Autodesk Fusion 360 part; units mm, degrees
(part 5 of 15)
sketch "Sketch1" plane through (0, 0, 0) normal (0, 0, 1) x (1, 0, 0) in component "Component"
  spline S0 degree 5 poles (15.0052, -0.9615) (15.0053, -0.9615) (15.0055, -0.9615) (15.0058, -0.9615) (15.0063, -0.9616) (15.0071, -0.9616) (15.008, -0.9616) (15.0091, -0.9617) (15.0102, -0.9617) (15.0115, -0.9618) (15.0128, -0.9618) (15.0143, -0.9619) (15.0159, -0.9619) (15.0176, -0.9619) (15.0194, -0.962) (15.0213, -0.962) (15.0234, -0.962) (15.0255, -0.9621) (15.0277, -0.9621) (15.0301, -0.9621) (15.0325, -0.9621) (15.0351, -0.9621) (15.0377, -0.9621) (15.0404, -0.9621) (15.0433, -0.9621) (15.0462, -0.9621) (15.0492, -0.962) (15.0523, -0.962) (15.0555, -0.9619) (15.0588, -0.9619) (15.0622, -0.9618) (15.0657, -0.9617) (15.0693, -0.9616) (15.0729, -0.9615) (15.0767, -0.9614) (15.0805, -0.9612) (15.0844, -0.9611) (15.0884, -0.9609) (15.0925, -0.9607) (15.0967, -0.9606) (15.1009, -0.9603) (15.1053, -0.9601) (15.1097, -0.9599) (15.1142, -0.9596) (15.1187, -0.9594) (15.1234, -0.9591) (15.1281, -0.9588) (15.1329, -0.9585) (15.1378, -0.9581) (15.1427, -0.9578) (15.1477, -0.9574) (15.1528, -0.957) (15.158, -0.9566) (15.1633, -0.9562) (15.1686, -0.9558) (15.174, -0.9553) (15.1794, -0.9548) (15.1849, -0.9543) (15.1905, -0.9538) (15.1962, -0.9533) (15.2019, -0.9527) (15.2077, -0.9521) (15.2136, -0.9515) (15.2196, -0.9509) (15.2256, -0.9503) (15.2316, -0.9496) (15.2378, -0.9489) (15.244, -0.9482) (15.2502, -0.9475) (15.2565, -0.9467) (15.2629, -0.946) (15.2694, -0.9452) (15.2759, -0.9444) (15.2825, -0.9435) (15.2891, -0.9427) (15.2958, -0.9418) (15.3025, -0.9408) (15.3094, -0.9399) (15.3162, -0.9389) (15.3232, -0.938) (15.3301, -0.937) (15.3372, -0.9359) (15.3443, -0.9349) (15.3515, -0.9338) (15.3587, -0.9327) (15.3659, -0.9315) (15.3733, -0.9304) (15.3807, -0.9292) (15.3881, -0.928) (15.3956, -0.9267) (15.4031, -0.9255) (15.4107, -0.9242) (15.4184, -0.9229) (15.4261, -0.9215) (15.4338, -0.9202) (15.4417, -0.9188) (15.4495, -0.9173) (15.4574, -0.9159) (15.4654, -0.9144) (15.4734, -0.9129) (15.4815, -0.9114) (15.4896, -0.9098) (15.4977, -0.9082) (15.5059, -0.9066) (15.5142, -0.905) (15.5225, -0.9033) (15.5309, -0.9016) (15.5393, -0.8999) (15.5477, -0.8981) (15.5562, -0.8963) (15.5648, -0.8945) (15.5733, -0.8927) (15.582, -0.8908) (15.5907, -0.8889) (15.5994, -0.887) (15.6081, -0.885) (15.617, -0.883) (15.6258, -0.881) (15.6347, -0.879) (15.6437, -0.8769) (15.6527, -0.8748) (15.6617, -0.8726) (15.6708, -0.8705) (15.6799, -0.8683) (15.689, -0.866) (15.6982, -0.8638) (15.7075, -0.8615) (15.7168, -0.8592) (15.7261, -0.8568) (15.7354, -0.8544) (15.7448, -0.852) (15.7543, -0.8496) (15.7638, -0.8471) (15.7733, -0.8446) (15.7829, -0.8421) (15.7925, -0.8395) (15.8021, -0.8369) (15.8118, -0.8343) (15.8215, -0.8316) (15.8313, -0.8289) (15.841, -0.8262) (15.8509, -0.8235) (15.8607, -0.8207) (15.8706, -0.8178) (15.8806, -0.815) (15.8906, -0.8121) (15.9006, -0.8092) (15.9106, -0.8063) (15.9207, -0.8033) (15.9308, -0.8003) (15.941, -0.7972) (15.9512, -0.7941) (15.9614, -0.791) (15.9716, -0.7879) (15.9819, -0.7847) (15.9923, -0.7815) (16.0026, -0.7783) (16.013, -0.775) (16.0234, -0.7717) (16.0339, -0.7683) (16.0444, -0.765) (16.0549, -0.7616) (16.0655, -0.7581) (16.0761, -0.7547) (16.0867, -0.7512) (16.0973, -0.7476) (16.108, -0.744) (16.1187, -0.7404) (16.1295, -0.7368) (16.1402, -0.7331) (16.151, -0.7294) (16.1619, -0.7257) (16.1727, -0.7219) (16.1836, -0.7181) (16.1946, -0.7143) (16.2055, -0.7104) (16.2165, -0.7065) (16.2275, -0.7025) (16.2385, -0.6986) (16.2496, -0.6946) (16.2607, -0.6905) (16.2718, -0.6864) (16.283, -0.6823) (16.2942, -0.6782) (16.3054, -0.674) (16.3166, -0.6698) (16.3279, -0.6655) (16.3391, -0.6612) (16.3505, -0.6569) (16.3618, -0.6526) (16.3732, -0.6482) (16.3846, -0.6438) (16.396, -0.6393) (16.4074, -0.6348) (16.4189, -0.6303) (16.4304, -0.6257) (16.4419, -0.6211) (16.4535, -0.6165) (16.465, -0.6118) (16.4766, -0.6071) (16.4882, -0.6024) (16.4999, -0.5976) (16.5116, -0.5928) (16.5233, -0.588) (16.535, -0.5831) (16.5467, -0.5782) (16.5585, -0.5732) (16.5703, -0.5683) (16.5821, -0.5632) (16.5939, -0.5582) (16.6057, -0.5531) (16.6176, -0.548) (16.6295, -0.5428) (16.6414, -0.5376) (16.6534, -0.5324) (16.6653, -0.5271) (16.6773, -0.5218) (16.6893, -0.5165) (16.7014, -0.5111) (16.7134, -0.5057) (16.7255, -0.5003) (16.7376, -0.4948) (16.7497, -0.4893) (16.7618, -0.4837) (16.774, -0.4782) (16.7861, -0.4725) (16.7983, -0.4669) (16.8105, -0.4612) (16.8228, -0.4555) (16.835, -0.4497) (16.8473, -0.4439) (16.8596, -0.4381) (16.8719, -0.4322) (16.8842, -0.4263) (16.8965, -0.4203) (16.9089, -0.4144) (16.9213, -0.4084) (16.9337, -0.4023) (16.9461, -0.3962) (16.9585, -0.3901) (16.971, -0.3839) (16.981, -0.379) (16.9884, -0.3753) (16.9934, -0.3728) (16.9959, -0.3715) knots 0 0 0 0 0 0 0.00416667 0.00833333 0.0125 0.01666667 0.02083333 0.025 0.02916667 0.03333333 0.0375 0.04166667 0.04583333 0.05 0.05416667 0.05833333 0.0625 0.06666667 0.07083333 0.075 0.07916667 0.08333333 0.0875 0.09166667 0.09583333 0.1 0.10416667 0.10833333 0.1125 0.11666667 0.12083333 0.125 0.12916667 0.13333333 0.1375 0.14166667 0.14583333 0.15 0.15416667 0.15833333 0.1625 0.16666667 0.17083333 0.175 0.17916667 0.18333333 0.1875 0.19166667 0.19583333 0.2 0.20416667 0.20833333 0.2125 0.21666667 0.22083333 0.225 0.22916667 0.23333333 0.2375 0.24166667 0.24583333 0.25 0.25416667 0.25833333 0.2625 0.26666667 0.27083333 0.275 0.27916667 0.28333333 0.2875 0.29166667 0.29583333 0.3 0.30416667 0.30833333 0.3125 0.31666667 0.32083333 0.325 0.32916667 0.33333333 0.3375 0.34166667 0.34583333 0.35 0.35416667 0.35833333 0.3625 0.36666667 0.37083333 0.375 0.37916667 0.38333333 0.3875 0.39166667 0.39583333 0.4 0.40416667 0.40833333 0.4125 0.41666667 0.42083333 0.425 0.42916667 0.43333333 0.4375 0.44166667 0.44583333 0.45 0.45416667 0.45833333 0.4625 0.46666667 0.47083333 0.475 0.47916667 0.48333333 0.4875 0.49166667 0.49583333 0.5 0.50416667 0.50833333 0.5125 0.51666667 0.52083333 0.525 0.52916667 0.53333333 0.5375 0.54166667 0.54583333 0.55 0.55416667 0.55833333 0.5625 0.56666667 0.57083333 0.575 0.57916667 0.58333333 0.5875 0.59166667 0.59583333 0.6 0.60416667 0.60833333 0.6125 0.61666667 0.62083333 0.625 0.62916667 0.63333333 0.6375 0.64166667 0.64583333 0.65 0.65416667 0.65833333 0.6625 0.66666667 0.67083333 0.675 0.67916667 0.68333333 0.6875 0.69166667 0.69583333 0.7 0.70416667 0.70833333 0.7125 0.71666667 0.72083333 0.725 0.72916667 0.73333333 0.7375 0.74166667 0.74583333 0.75 0.75416667 0.75833333 0.7625 0.76666667 0.77083333 0.775 0.77916667 0.78333333 0.7875 0.79166667 0.79583333 0.8 0.80416667 0.80833333 0.8125 0.81666667 0.82083333 0.825 0.82916667 0.83333333 0.8375 0.84166667 0.84583333 0.85 0.85416667 0.85833333 0.8625 0.86666667 0.87083333 0.875 0.87916667 0.88333333 0.8875 0.89166667 0.89583333 0.9 0.90416667 0.90833333 0.9125 0.91666667 0.92083333 0.925 0.92916667 0.93333333 0.9375 0.94166667 0.94583333 0.95 0.95416667 0.95833333 0.9625 0.96666667 0.97083333 0.975 0.97916667 0.98333333 0.9875 0.99166667 0.99583333 1 1 1 1 1 1
  spline S1 degree 5 poles (15.0052, 0.9615) (15.0053, 0.9615) (15.0055, 0.9615) (15.0058, 0.9615) (15.0063, 0.9616) (15.0071, 0.9616) (15.008, 0.9616) (15.0091, 0.9617) (15.0102, 0.9617) (15.0115, 0.9618) (15.0128, 0.9618) (15.0143, 0.9619) (15.0159, 0.9619) (15.0176, 0.9619) (15.0194, 0.962) (15.0213, 0.962) (15.0234, 0.962) (15.0255, 0.9621) (15.0277, 0.9621) (15.0301, 0.9621) (15.0325, 0.9621) (15.0351, 0.9621) (15.0377, 0.9621) (15.0404, 0.9621) (15.0433, 0.9621) (15.0462, 0.9621) (15.0492, 0.962) (15.0523, 0.962) (15.0555, 0.9619) (15.0588, 0.9619) (15.0622, 0.9618) (15.0657, 0.9617) (15.0693, 0.9616) (15.0729, 0.9615) (15.0767, 0.9614) (15.0805, 0.9612) (15.0844, 0.9611) (15.0884, 0.9609) (15.0925, 0.9607) (15.0967, 0.9606) (15.1009, 0.9603) (15.1053, 0.9601) (15.1097, 0.9599) (15.1142, 0.9596) (15.1187, 0.9594) (15.1234, 0.9591) (15.1281, 0.9588) (15.1329, 0.9585) (15.1378, 0.9581) (15.1427, 0.9578) (15.1477, 0.9574) (15.1528, 0.957) (15.158, 0.9566) (15.1633, 0.9562) (15.1686, 0.9558) (15.174, 0.9553) (15.1794, 0.9548) (15.1849, 0.9543) (15.1905, 0.9538) (15.1962, 0.9533) (15.2019, 0.9527) (15.2077, 0.9521) (15.2136, 0.9515) (15.2196, 0.9509) (15.2256, 0.9503) (15.2316, 0.9496) (15.2378, 0.9489) (15.244, 0.9482) (15.2502, 0.9475) (15.2565, 0.9467) (15.2629, 0.946) (15.2694, 0.9452) (15.2759, 0.9444) (15.2825, 0.9435) (15.2891, 0.9427) (15.2958, 0.9418) (15.3025, 0.9408) (15.3094, 0.9399) (15.3162, 0.9389) (15.3232, 0.938) (15.3301, 0.937) (15.3372, 0.9359) (15.3443, 0.9349) (15.3515, 0.9338) (15.3587, 0.9327) (15.3659, 0.9315) (15.3733, 0.9304) (15.3807, 0.9292) (15.3881, 0.928) (15.3956, 0.9267) (15.4031, 0.9255) (15.4107, 0.9242) (15.4184, 0.9229) (15.4261, 0.9215) (15.4338, 0.9202) (15.4417, 0.9188) (15.4495, 0.9173) (15.4574, 0.9159) (15.4654, 0.9144) (15.4734, 0.9129) (15.4815, 0.9114) (15.4896, 0.9098) (15.4977, 0.9082) (15.5059, 0.9066) (15.5142, 0.905) (15.5225, 0.9033) (15.5309, 0.9016) (15.5393, 0.8999) (15.5477, 0.8981) (15.5562, 0.8963) (15.5648, 0.8945) (15.5733, 0.8927) (15.582, 0.8908) (15.5907, 0.8889) (15.5994, 0.887) (15.6081, 0.885) (15.617, 0.883) (15.6258, 0.881) (15.6347, 0.879) (15.6437, 0.8769) (15.6527, 0.8748) (15.6617, 0.8726) (15.6708, 0.8705) (15.6799, 0.8683) (15.689, 0.866) (15.6982, 0.8638) (15.7075, 0.8615) (15.7168, 0.8592) (15.7261, 0.8568) (15.7354, 0.8544) (15.7448, 0.852) (15.7543, 0.8496) (15.7638, 0.8471) (15.7733, 0.8446) (15.7829, 0.8421) (15.7925, 0.8395) (15.8021, 0.8369) (15.8118, 0.8343) (15.8215, 0.8316) (15.8313, 0.8289) (15.841, 0.8262) (15.8509, 0.8235) (15.8607, 0.8207) (15.8706, 0.8178) (15.8806, 0.815) (15.8906, 0.8121) (15.9006, 0.8092) (15.9106, 0.8063) (15.9207, 0.8033) (15.9308, 0.8003) (15.941, 0.7972) (15.9512, 0.7941) (15.9614, 0.791) (15.9716, 0.7879) (15.9819, 0.7847) (15.9923, 0.7815) (16.0026, 0.7783) (16.013, 0.775) (16.0234, 0.7717) (16.0339, 0.7683) (16.0444, 0.765) (16.0549, 0.7616) (16.0655, 0.7581) (16.0761, 0.7547) (16.0867, 0.7512) (16.0973, 0.7476) (16.108, 0.744) (16.1187, 0.7404) (16.1295, 0.7368) (16.1402, 0.7331) (16.151, 0.7294) (16.1619, 0.7257) (16.1727, 0.7219) (16.1836, 0.7181) (16.1946, 0.7143) (16.2055, 0.7104) (16.2165, 0.7065) (16.2275, 0.7025) (16.2385, 0.6986) (16.2496, 0.6946) (16.2607, 0.6905) (16.2718, 0.6864) (16.283, 0.6823) (16.2942, 0.6782) (16.3054, 0.674) (16.3166, 0.6698) (16.3279, 0.6655) (16.3391, 0.6612) (16.3505, 0.6569) (16.3618, 0.6526) (16.3732, 0.6482) (16.3846, 0.6438) (16.396, 0.6393) (16.4074, 0.6348) (16.4189, 0.6303) (16.4304, 0.6257) (16.4419, 0.6211) (16.4535, 0.6165) (16.465, 0.6118) (16.4766, 0.6071) (16.4882, 0.6024) (16.4999, 0.5976) (16.5116, 0.5928) (16.5233, 0.588) (16.535, 0.5831) (16.5467, 0.5782) (16.5585, 0.5732) (16.5703, 0.5683) (16.5821, 0.5632) (16.5939, 0.5582) (16.6057, 0.5531) (16.6176, 0.548) (16.6295, 0.5428) (16.6414, 0.5376) (16.6534, 0.5324) (16.6653, 0.5271) (16.6773, 0.5218) (16.6893, 0.5165) (16.7014, 0.5111) (16.7134, 0.5057) (16.7255, 0.5003) (16.7376, 0.4948) (16.7497, 0.4893) (16.7618, 0.4837) (16.774, 0.4782) (16.7861, 0.4725) (16.7983, 0.4669) (16.8105, 0.4612) (16.8228, 0.4555) (16.835, 0.4497) (16.8473, 0.4439) (16.8596, 0.4381) (16.8719, 0.4322) (16.8842, 0.4263) (16.8965, 0.4203) (16.9089, 0.4144) (16.9213, 0.4084) (16.9337, 0.4023) (16.9461, 0.3962) (16.9585, 0.3901) (16.971, 0.3839) (16.981, 0.379) (16.9884, 0.3753) (16.9934, 0.3728) (16.9959, 0.3715) knots 0 0 0 0 0 0 0.00416667 0.00833333 0.0125 0.01666667 0.02083333 0.025 0.02916667 0.03333333 0.0375 0.04166667 0.04583333 0.05 0.05416667 0.05833333 0.0625 0.06666667 0.07083333 0.075 0.07916667 0.08333333 0.0875 0.09166667 0.09583333 0.1 0.10416667 0.10833333 0.1125 0.11666667 0.12083333 0.125 0.12916667 0.13333333 0.1375 0.14166667 0.14583333 0.15 0.15416667 0.15833333 0.1625 0.16666667 0.17083333 0.175 0.17916667 0.18333333 0.1875 0.19166667 0.19583333 0.2 0.20416667 0.20833333 0.2125 0.21666667 0.22083333 0.225 0.22916667 0.23333333 0.2375 0.24166667 0.24583333 0.25 0.25416667 0.25833333 0.2625 0.26666667 0.27083333 0.275 0.27916667 0.28333333 0.2875 0.29166667 0.29583333 0.3 0.30416667 0.30833333 0.3125 0.31666667 0.32083333 0.325 0.32916667 0.33333333 0.3375 0.34166667 0.34583333 0.35 0.35416667 0.35833333 0.3625 0.36666667 0.37083333 0.375 0.37916667 0.38333333 0.3875 0.39166667 0.39583333 0.4 0.40416667 0.40833333 0.4125 0.41666667 0.42083333 0.425 0.42916667 0.43333333 0.4375 0.44166667 0.44583333 0.45 0.45416667 0.45833333 0.4625 0.46666667 0.47083333 0.475 0.47916667 0.48333333 0.4875 0.49166667 0.49583333 0.5 0.50416667 0.50833333 0.5125 0.51666667 0.52083333 0.525 0.52916667 0.53333333 0.5375 0.54166667 0.54583333 0.55 0.55416667 0.55833333 0.5625 0.56666667 0.57083333 0.575 0.57916667 0.58333333 0.5875 0.59166667 0.59583333 0.6 0.60416667 0.60833333 0.6125 0.61666667 0.62083333 0.625 0.62916667 0.63333333 0.6375 0.64166667 0.64583333 0.65 0.65416667 0.65833333 0.6625 0.66666667 0.67083333 0.675 0.67916667 0.68333333 0.6875 0.69166667 0.69583333 0.7 0.70416667 0.70833333 0.7125 0.71666667 0.72083333 0.725 0.72916667 0.73333333 0.7375 0.74166667 0.74583333 0.75 0.75416667 0.75833333 0.7625 0.76666667 0.77083333 0.775 0.77916667 0.78333333 0.7875 0.79166667 0.79583333 0.8 0.80416667 0.80833333 0.8125 0.81666667 0.82083333 0.825 0.82916667 0.83333333 0.8375 0.84166667 0.84583333 0.85 0.85416667 0.85833333 0.8625 0.86666667 0.87083333 0.875 0.87916667 0.88333333 0.8875 0.89166667 0.89583333 0.9 0.90416667 0.90833333 0.9125 0.91666667 0.92083333 0.925 0.92916667 0.93333333 0.9375 0.94166667 0.94583333 0.95 0.95416667 0.95833333 0.9625 0.96666667 0.97083333 0.975 0.97916667 0.98333333 0.9875 0.99166667 0.99583333 1 1 1 1 1 1
  spline S2 degree 5 poles (15.0043, -0.9615) (15.0043, -0.9615) (15.0044, -0.9615) (15.0045, -0.9615) (15.0047, -0.9615) (15.0048, -0.9615) (15.005, -0.9615) (15.0051, -0.9615) (15.0051, -0.9615) (15.0052, -0.9615) knots 0 0 0 0 0 0 0.2 0.4 0.6 0.8 1 1 1 1 1 1
  spline S3 degree 5 poles (15.0043, 0.9615) (15.0043, 0.9615) (15.0044, 0.9615) (15.0045, 0.9615) (15.0047, 0.9615) (15.0048, 0.9615) (15.005, 0.9615) (15.0051, 0.9615) (15.0051, 0.9615) (15.0052, 0.9615) knots 0 0 0 0 0 0 0.2 0.4 0.6 0.8 1 1 1 1 1 1
  line L0 (0, 0) -> (15.0043, -0.9615)
  line L1 (0, 0) -> (15.0043, 0.9615)
  arc A0 (16.9959, -0.3715) -> (16.9959, 0.3715) centre (0, 0) ccw
  point P0 (15.0078, -0.9616)
  point P1 (15.0121, -0.9618)
  point P2 (15.0182, -0.962)
  point P3 (15.0261, -0.9621)
  point P4 (15.0357, -0.9621)
  point P5 (15.047, -0.9621)
  point P6 (15.0601, -0.9618)
  point P7 (15.0749, -0.9614)
  point P8 (15.0915, -0.9608)
  point P9 (15.1097, -0.9599)
  point P10 (15.1298, -0.9587)
  point P11 (15.1515, -0.9571)
  point P12 (15.175, -0.9552)
  point P13 (15.2001, -0.9529)
  point P14 (15.227, -0.9501)
  point P15 (15.2556, -0.9469)
  point P16 (15.2859, -0.9431)
  point P17 (15.3179, -0.9387)
  point P18 (15.3515, -0.9338)
  point P19 (15.3868, -0.9282)
  point P20 (15.4238, -0.9219)
  point P21 (15.4624, -0.915)
  point P22 (15.5026, -0.9073)
  point P23 (15.5445, -0.8988)
  point P24 (15.588, -0.8895)
  point P25 (15.6331, -0.8793)
  point P26 (15.6797, -0.8683)
  point P27 (15.728, -0.8563)
  point P28 (15.7777, -0.8434)
  point P29 (15.8291, -0.8295)
  point P30 (15.8819, -0.8146)
  point P31 (15.9363, -0.7986)
  point P32 (15.9922, -0.7815)
  point P33 (16.0495, -0.7633)
  point P34 (16.1083, -0.7439)
  point P35 (16.1685, -0.7234)
  point P36 (16.2302, -0.7016)
  point P37 (16.2932, -0.6785)
  point P38 (16.3576, -0.6542)
  point P39 (16.4234, -0.6285)
  point P40 (16.4905, -0.6014)
  point P41 (16.559, -0.573)
  point P42 (16.6287, -0.5432)
  point P43 (16.6997, -0.5119)
  point P44 (16.772, -0.4791)
  point P45 (16.8454, -0.4448)
  point P46 (16.9201, -0.4089)
  point P47 (15.0078, 0.9616)
  point P48 (15.0121, 0.9618)
  point P49 (15.0182, 0.962)
  point P50 (15.0261, 0.9621)
  point P51 (15.0357, 0.9621)
  point P52 (15.047, 0.9621)
  point P53 (15.0601, 0.9618)
  point P54 (15.0749, 0.9614)
  point P55 (15.0915, 0.9608)
  point P56 (15.1097, 0.9599)
  point P57 (15.1298, 0.9587)
  point P58 (15.1515, 0.9571)
  point P59 (15.175, 0.9552)
  point P60 (15.2001, 0.9529)
  point P61 (15.227, 0.9501)
  point P62 (15.2556, 0.9469)
  point P63 (15.2859, 0.9431)
  point P64 (15.3179, 0.9387)
  point P65 (15.3515, 0.9338)
  point P66 (15.3868, 0.9282)
  point P67 (15.4238, 0.9219)
  point P68 (15.4624, 0.915)
  point P69 (15.5026, 0.9073)
  point P70 (15.5445, 0.8988)
  point P71 (15.588, 0.8895)
  point P72 (15.6331, 0.8793)
  point P73 (15.6797, 0.8683)
  point P74 (15.728, 0.8563)
  point P75 (15.7777, 0.8434)
  point P76 (15.8291, 0.8295)
  point P77 (15.8819, 0.8146)
  point P78 (15.9363, 0.7986)
  point P79 (15.9922, 0.7815)
  point P80 (16.0495, 0.7633)
  point P81 (16.1083, 0.7439)
  point P82 (16.1685, 0.7234)
  point P83 (16.2302, 0.7016)
  point P84 (16.2932, 0.6785)
  point P85 (16.3576, 0.6542)
  point P86 (16.4234, 0.6285)
  point P87 (16.4905, 0.6014)
  point P88 (16.559, 0.573)
  point P89 (16.6287, 0.5432)
  point P90 (16.6997, 0.5119)
  point P91 (16.772, 0.4791)
  point P92 (16.8454, 0.4448)
  point P93 (16.9201, 0.4089)
sketch "Sketch2" plane through (0, 0, 0) normal (0, 0, 1) x (1, 0, 0) in component "Component"
  circle A0 centre (0, 0) radius 14.75
extrude "Extrude1" add sketch "Sketch2" along normal blind 10 makes body 1 in component "Component"
extrude "Extrude2" add sketch "Sketch1" along normal blind 10 separate body makes body 2 in component "Component"
pattern_circular "C-Pattern1" count 32 over 360 about axis through (0, 0, 1.75) along (0, 0, 1) of "Extrude2" makes body 3 at (4.8431, 1.2901, 3.3333) makes body 4 at (4.7436, 1.618, 3.3333) makes body 5 at (4.3368, 2.5123, 3.3333) makes body 6 at (3.7634, 3.3101, 6.6667) makes body 7 at (3.0453, 3.9807, 3.3333) makes body 8 at (2.2102, 4.4983, 6.6667) makes body 9 at (1.2901, 4.8431, 3.3333) makes body 10 at (0.3205, 5.0017, 3.3333) makes body 11 at (-1.2901, 4.8431, 3.3333) makes body 12 at (-1.618, 4.7436, 6.6667) makes body 13 at (-2.5123, 4.3368, 3.3333) makes body 14 at (-3.3101, 3.7634, 3.3333) makes body 15 at (-3.9807, 3.0453, 3.3333) makes body 16 at (-4.7436, 1.618, 3.3333) makes body 17 at (-4.8431, 1.2901, 3.3333) makes body 18 at (-5.0017, 0.3205, 6.6667) makes body 19 at (-4.9681, -0.6614, 6.6667) makes body 20 at (-4.7436, -1.618, 6.6667) makes body 21 at (-4.3368, -2.5123, 3.3333) makes body 22 at (-3.7634, -3.3101, 3.3333) makes body 23 at (-3.0453, -3.9807, 3.3333) makes body 24 at (-2.2102, -4.4983, 3.3333) makes body 25 at (-1.2901, -4.8431, 3.3333) makes body 26 at (-0.3205, -5.0017, 6.6667) makes body 27 at (0.6614, -4.9681, 6.6667) makes body 28 at (1.618, -4.7436, 6.6667) makes body 29 at (2.5123, -4.3368, 3.3333) makes body 30 at (3.3101, -3.7634, 6.6667) makes body 31 at (4.3368, -2.5123, 3.3333) makes body 32 at (4.7436, -1.618, 6.6667) makes body 33 at (4.8431, -1.2901, 3.3333) in component "Component"
combine "Combine1" operation add target body 1 tool bodies 2 3 4 5 6 7 8 9 10 11 12 13 14 15 16 17 18 19 20 21 22 23 24 25 26 27 28 29 30 31 32 33 in component "Component"
sketch "Sketch3" plane through (0, 0, 0) normal (0, 0, 1) x (1, 0, 0) in component "Component"
  line L0 (0, 0) -> (47.0171, 0) construction
  line L1 (47.0171, 0) -> (47.0171, 3) construction
  line L2 (47.0171, 3) -> (0, 3) construction
  line L3 (0, 3) -> (0, 0) construction
  constraint perpendicular L0 L1
  constraint parallel L0 L2
  constraint parallel L1 L3
sketch "Sketch1 (2)" plane through (0, 0, 10) normal (0, 0, 1) x (-1, 0, 0)
  arc A0 (-14.621, 1.9466) -> (-14.7198, 0.9432) centre (0, 0) ccw
  line L0 (-14.7198, 0.9432) -> (-15.0043, 0.9615)
  line L1 (-15.0043, 0.9615) -> (-15.0052, 0.9615)
  spline S0 degree 5 poles (-15.0052, 0.9615) (-15.0053, 0.9615) (-15.0055, 0.9615) (-15.0058, 0.9615) (-15.0063, 0.9616) (-15.0071, 0.9616) (-15.008, 0.9616) (-15.0091, 0.9617) (-15.0102, 0.9617) (-15.0115, 0.9618) (-15.0128, 0.9618) (-15.0143, 0.9619) (-15.0159, 0.9619) (-15.0176, 0.9619) (-15.0194, 0.962) (-15.0213, 0.962) (-15.0234, 0.962) (-15.0255, 0.9621) (-15.0277, 0.9621) (-15.0301, 0.9621) (-15.0325, 0.9621) (-15.0351, 0.9621) (-15.0377, 0.9621) (-15.0404, 0.9621) (-15.0433, 0.9621) (-15.0462, 0.9621) (-15.0492, 0.962) (-15.0523, 0.962) (-15.0555, 0.9619) (-15.0588, 0.9619) (-15.0622, 0.9618) (-15.0657, 0.9617) (-15.0693, 0.9616) (-15.0729, 0.9615) (-15.0767, 0.9614) (-15.0805, 0.9612) (-15.0844, 0.9611) (-15.0884, 0.9609) (-15.0925, 0.9607) (-15.0967, 0.9606) (-15.1009, 0.9603) (-15.1053, 0.9601) (-15.1097, 0.9599) (-15.1142, 0.9596) (-15.1187, 0.9594) (-15.1234, 0.9591) (-15.1281, 0.9588) (-15.1329, 0.9585) (-15.1378, 0.9581) (-15.1427, 0.9578) (-15.1477, 0.9574) (-15.1528, 0.957) (-15.158, 0.9566) (-15.1633, 0.9562) (-15.1686, 0.9558) (-15.174, 0.9553) (-15.1794, 0.9548) (-15.1849, 0.9543) (-15.1905, 0.9538) (-15.1962, 0.9533) (-15.2019, 0.9527) (-15.2077, 0.9521) (-15.2136, 0.9515) (-15.2196, 0.9509) (-15.2256, 0.9503) (-15.2316, 0.9496) (-15.2378, 0.9489) (-15.244, 0.9482) (-15.2502, 0.9475) (-15.2565, 0.9467) (-15.2629, 0.946) (-15.2694, 0.9452) (-15.2759, 0.9444) (-15.2825, 0.9435) (-15.2891, 0.9427) (-15.2958, 0.9418) (-15.3025, 0.9408) (-15.3094, 0.9399) (-15.3162, 0.9389) (-15.3232, 0.938) (-15.3301, 0.937) (-15.3372, 0.9359) (-15.3443, 0.9349) (-15.3515, 0.9338) (-15.3587, 0.9327) (-15.3659, 0.9315) (-15.3733, 0.9304) (-15.3807, 0.9292) (-15.3881, 0.928) (-15.3956, 0.9267) (-15.4031, 0.9255) (-15.4107, 0.9242) (-15.4184, 0.9229) (-15.4261, 0.9215) (-15.4338, 0.9202) (-15.4417, 0.9188) (-15.4495, 0.9173) (-15.4574, 0.9159) (-15.4654, 0.9144) (-15.4734, 0.9129) (-15.4815, 0.9114) (-15.4896, 0.9098) (-15.4977, 0.9082) (-15.5059, 0.9066) (-15.5142, 0.905) (-15.5225, 0.9033) (-15.5309, 0.9016) (-15.5393, 0.8999) (-15.5477, 0.8981) (-15.5562, 0.8963) (-15.5648, 0.8945) (-15.5733, 0.8927) (-15.582, 0.8908) (-15.5907, 0.8889) (-15.5994, 0.887) (-15.6081, 0.885) (-15.617, 0.883) (-15.6258, 0.881) (-15.6347, 0.879) (-15.6437, 0.8769) (-15.6527, 0.8748) (-15.6617, 0.8726) (-15.6708, 0.8705) (-15.6799, 0.8683) (-15.689, 0.866) (-15.6982, 0.8638) (-15.7075, 0.8615) (-15.7168, 0.8592) (-15.7261, 0.8568) (-15.7354, 0.8544) (-15.7448, 0.852) (-15.7543, 0.8496) (-15.7638, 0.8471) (-15.7733, 0.8446) (-15.7829, 0.8421) (-15.7925, 0.8395) (-15.8021, 0.8369) (-15.8118, 0.8343) (-15.8215, 0.8316) (-15.8313, 0.8289) (-15.841, 0.8262) (-15.8509, 0.8235) (-15.8607, 0.8207) (-15.8706, 0.8178) (-15.8806, 0.815) (-15.8906, 0.8121) (-15.9006, 0.8092) (-15.9106, 0.8063) (-15.9207, 0.8033) (-15.9308, 0.8003) (-15.941, 0.7972) (-15.9512, 0.7941) (-15.9614, 0.791) (-15.9716, 0.7879) (-15.9819, 0.7847) (-15.9923, 0.7815) (-16.0026, 0.7783) (-16.013, 0.775) (-16.0234, 0.7717) (-16.0339, 0.7683) (-16.0444, 0.765) (-16.0549, 0.7616) (-16.0655, 0.7581) (-16.0761, 0.7547) (-16.0867, 0.7512) (-16.0973, 0.7476) (-16.108, 0.744) (-16.1187, 0.7404) (-16.1295, 0.7368) (-16.1402, 0.7331) (-16.151, 0.7294) (-16.1619, 0.7257) (-16.1727, 0.7219) (-16.1836, 0.7181) (-16.1946, 0.7143) (-16.2055, 0.7104) (-16.2165, 0.7065) (-16.2275, 0.7025) (-16.2385, 0.6986) (-16.2496, 0.6946) (-16.2607, 0.6905) (-16.2718, 0.6864) (-16.283, 0.6823) (-16.2942, 0.6782) (-16.3054, 0.674) (-16.3166, 0.6698) (-16.3279, 0.6655) (-16.3391, 0.6612) (-16.3505, 0.6569) (-16.3618, 0.6526) (-16.3732, 0.6482) (-16.3846, 0.6438) (-16.396, 0.6393) (-16.4074, 0.6348) (-16.4189, 0.6303) (-16.4304, 0.6257) (-16.4419, 0.6211) (-16.4535, 0.6165) (-16.465, 0.6118) (-16.4766, 0.6071) (-16.4882, 0.6024) (-16.4999, 0.5976) (-16.5116, 0.5928) (-16.5233, 0.588) (-16.535, 0.5831) (-16.5467, 0.5782) (-16.5585, 0.5732) (-16.5703, 0.5683) (-16.5821, 0.5632) (-16.5939, 0.5582) (-16.6057, 0.5531) (-16.6176, 0.548) (-16.6295, 0.5428) (-16.6414, 0.5376) (-16.6534, 0.5324) (-16.6653, 0.5271) (-16.6773, 0.5218) (-16.6893, 0.5165) (-16.7014, 0.5111) (-16.7134, 0.5057) (-16.7255, 0.5003) (-16.7376, 0.4948) (-16.7497, 0.4893) (-16.7618, 0.4837) (-16.774, 0.4782) (-16.7861, 0.4725) (-16.7983, 0.4669) (-16.8105, 0.4612) (-16.8228, 0.4555) (-16.835, 0.4497) (-16.8473, 0.4439) (-16.8596, 0.4381) (-16.8719, 0.4322) (-16.8842, 0.4263) (-16.8965, 0.4203) (-16.9089, 0.4144) (-16.9213, 0.4084) (-16.9337, 0.4023) (-16.9461, 0.3962) (-16.9585, 0.3901) (-16.971, 0.3839) (-16.981, 0.379) (-16.9884, 0.3753) (-16.9934, 0.3728) (-16.9959, 0.3715) knots 0 0 0 0 0 0 0.00416667 0.00833333 0.0125 0.01666667 0.02083333 0.025 0.02916667 0.03333333 0.0375 0.04166667 0.04583333 0.05 0.05416667 0.05833333 0.0625 0.06666667 0.07083333 0.075 0.07916667 0.08333333 0.0875 0.09166667 0.09583333 0.1 0.10416667 0.10833333 0.1125 0.11666667 0.12083333 0.125 0.12916667 0.13333333 0.1375 0.14166667 0.14583333 0.15 0.15416667 0.15833333 0.1625 0.16666667 0.17083333 0.175 0.17916667 0.18333333 0.1875 0.19166667 0.19583333 0.2 0.20416667 0.20833333 0.2125 0.21666667 0.22083333 0.225 0.22916667 0.23333333 0.2375 0.24166667 0.24583333 0.25 0.25416667 0.25833333 0.2625 0.26666667 0.27083333 0.275 0.27916667 0.28333333 0.2875 0.29166667 0.29583333 0.3 0.30416667 0.30833333 0.3125 0.31666667 0.32083333 0.325 0.32916667 0.33333333 0.3375 0.34166667 0.34583333 0.35 0.35416667 0.35833333 0.3625 0.36666667 0.37083333 0.375 0.37916667 0.38333333 0.3875 0.39166667 0.39583333 0.4 0.40416667 0.40833333 0.4125 0.41666667 0.42083333 0.425 0.42916667 0.43333333 0.4375 0.44166667 0.44583333 0.45 0.45416667 0.45833333 0.4625 0.46666667 0.47083333 0.475 0.47916667 0.48333333 0.4875 0.49166667 0.49583333 0.5 0.50416667 0.50833333 0.5125 0.51666667 0.52083333 0.525 0.52916667 0.53333333 0.5375 0.54166667 0.54583333 0.55 0.55416667 0.55833333 0.5625 0.56666667 0.57083333 0.575 0.57916667 0.58333333 0.5875 0.59166667 0.59583333 0.6 0.60416667 0.60833333 0.6125 0.61666667 0.62083333 0.625 0.62916667 0.63333333 0.6375 0.64166667 0.64583333 0.65 0.65416667 0.65833333 0.6625 0.66666667 0.67083333 0.675 0.67916667 0.68333333 0.6875 0.69166667 0.69583333 0.7 0.70416667 0.70833333 0.7125 0.71666667 0.72083333 0.725 0.72916667 0.73333333 0.7375 0.74166667 0.74583333 0.75 0.75416667 0.75833333 0.7625 0.76666667 0.77083333 0.775 0.77916667 0.78333333 0.7875 0.79166667 0.79583333 0.8 0.80416667 0.80833333 0.8125 0.81666667 0.82083333 0.825 0.82916667 0.83333333 0.8375 0.84166667 0.84583333 0.85 0.85416667 0.85833333 0.8625 0.86666667 0.87083333 0.875 0.87916667 0.88333333 0.8875 0.89166667 0.89583333 0.9 0.90416667 0.90833333 0.9125 0.91666667 0.92083333 0.925 0.92916667 0.93333333 0.9375 0.94166667 0.94583333 0.95 0.95416667 0.95833333 0.9625 0.96666667 0.97083333 0.975 0.97916667 0.98333333 0.9875 0.99166667 0.99583333 1 1 1 1 1 1
  arc A1 (-16.9959, 0.3715) -> (-16.9959, -0.3715) centre (0, 0) ccw
  spline S1 degree 5 poles (-16.9959, -0.3715) (-16.9934, -0.3728) (-16.9884, -0.3753) (-16.981, -0.379) (-16.971, -0.3839) (-16.9585, -0.3901) (-16.9461, -0.3962) (-16.9337, -0.4023) (-16.9213, -0.4084) (-16.9089, -0.4144) (-16.8965, -0.4203) (-16.8842, -0.4263) (-16.8719, -0.4322) (-16.8596, -0.4381) (-16.8473, -0.4439) (-16.835, -0.4497) (-16.8228, -0.4555) (-16.8105, -0.4612) (-16.7983, -0.4669) (-16.7861, -0.4725) (-16.774, -0.4782) (-16.7618, -0.4837) (-16.7497, -0.4893) (-16.7376, -0.4948) (-16.7255, -0.5003) (-16.7134, -0.5057) (-16.7014, -0.5111) (-16.6893, -0.5165) (-16.6773, -0.5218) (-16.6653, -0.5271) (-16.6534, -0.5324) (-16.6414, -0.5376) (-16.6295, -0.5428) (-16.6176, -0.548) (-16.6057, -0.5531) (-16.5939, -0.5582) (-16.5821, -0.5632) (-16.5703, -0.5683) (-16.5585, -0.5732) (-16.5467, -0.5782) (-16.535, -0.5831) (-16.5233, -0.588) (-16.5116, -0.5928) (-16.4999, -0.5976) (-16.4882, -0.6024) (-16.4766, -0.6071) (-16.465, -0.6118) (-16.4535, -0.6165) (-16.4419, -0.6211) (-16.4304, -0.6257) (-16.4189, -0.6303) (-16.4074, -0.6348) (-16.396, -0.6393) (-16.3846, -0.6438) (-16.3732, -0.6482) (-16.3618, -0.6526) (-16.3505, -0.6569) (-16.3391, -0.6612) (-16.3279, -0.6655) (-16.3166, -0.6698) (-16.3054, -0.674) (-16.2942, -0.6782) (-16.283, -0.6823) (-16.2718, -0.6864) (-16.2607, -0.6905) (-16.2496, -0.6946) (-16.2385, -0.6986) (-16.2275, -0.7025) (-16.2165, -0.7065) (-16.2055, -0.7104) (-16.1946, -0.7143) (-16.1836, -0.7181) (-16.1727, -0.7219) (-16.1619, -0.7257) (-16.151, -0.7294) (-16.1402, -0.7331) (-16.1295, -0.7368) (-16.1187, -0.7404) (-16.108, -0.744) (-16.0973, -0.7476) (-16.0867, -0.7512) (-16.0761, -0.7547) (-16.0655, -0.7581) (-16.0549, -0.7616) (-16.0444, -0.765) (-16.0339, -0.7683) (-16.0234, -0.7717) (-16.013, -0.775) (-16.0026, -0.7783) (-15.9923, -0.7815) (-15.9819, -0.7847) (-15.9716, -0.7879) (-15.9614, -0.791) (-15.9512, -0.7941) (-15.941, -0.7972) (-15.9308, -0.8003) (-15.9207, -0.8033) (-15.9106, -0.8063) (-15.9006, -0.8092) (-15.8906, -0.8121) (-15.8806, -0.815) (-15.8706, -0.8178) (-15.8607, -0.8207) (-15.8509, -0.8235) (-15.841, -0.8262) (-15.8313, -0.8289) (-15.8215, -0.8316) (-15.8118, -0.8343) (-15.8021, -0.8369) (-15.7925, -0.8395) (-15.7829, -0.8421) (-15.7733, -0.8446) (-15.7638, -0.8471) (-15.7543, -0.8496) (-15.7448, -0.852) (-15.7354, -0.8544) (-15.7261, -0.8568) (-15.7168, -0.8592) (-15.7075, -0.8615) (-15.6982, -0.8638) (-15.689, -0.866) (-15.6799, -0.8683) (-15.6708, -0.8705) (-15.6617, -0.8726) (-15.6527, -0.8748) (-15.6437, -0.8769) (-15.6347, -0.879) (-15.6258, -0.881) (-15.617, -0.883) (-15.6081, -0.885) (-15.5994, -0.887) (-15.5907, -0.8889) (-15.582, -0.8908) (-15.5733, -0.8927) (-15.5648, -0.8945) (-15.5562, -0.8963) (-15.5477, -0.8981) (-15.5393, -0.8999) (-15.5309, -0.9016) (-15.5225, -0.9033) (-15.5142, -0.905) (-15.5059, -0.9066) (-15.4977, -0.9082) (-15.4896, -0.9098) (-15.4815, -0.9114) (-15.4734, -0.9129) (-15.4654, -0.9144) (-15.4574, -0.9159) (-15.4495, -0.9173) (-15.4417, -0.9188) (-15.4338, -0.9202) (-15.4261, -0.9215) (-15.4184, -0.9229) (-15.4107, -0.9242) (-15.4031, -0.9255) (-15.3956, -0.9267) (-15.3881, -0.928) (-15.3807, -0.9292) (-15.3733, -0.9304) (-15.3659, -0.9315) (-15.3587, -0.9327) (-15.3515, -0.9338) (-15.3443, -0.9349) (-15.3372, -0.9359) (-15.3301, -0.937) (-15.3232, -0.938) (-15.3162, -0.9389) (-15.3094, -0.9399) (-15.3025, -0.9408) (-15.2958, -0.9418) (-15.2891, -0.9427) (-15.2825, -0.9435) (-15.2759, -0.9444) (-15.2694, -0.9452) (-15.2629, -0.946) (-15.2565, -0.9467) (-15.2502, -0.9475) (-15.244, -0.9482) (-15.2378, -0.9489) (-15.2316, -0.9496) (-15.2256, -0.9503) (-15.2196, -0.9509) (-15.2136, -0.9515) (-15.2077, -0.9521) (-15.2019, -0.9527) (-15.1962, -0.9533) (-15.1905, -0.9538) (-15.1849, -0.9543) (-15.1794, -0.9548) (-15.174, -0.9553) (-15.1686, -0.9558) (-15.1633, -0.9562) (-15.158, -0.9566) (-15.1528, -0.957) (-15.1477, -0.9574) (-15.1427, -0.9578) (-15.1378, -0.9581) (-15.1329, -0.9585) (-15.1281, -0.9588) (-15.1234, -0.9591) (-15.1187, -0.9594) (-15.1142, -0.9596) (-15.1097, -0.9599) (-15.1053, -0.9601) (-15.1009, -0.9603) (-15.0967, -0.9606) (-15.0925, -0.9607) (-15.0884, -0.9609) (-15.0844, -0.9611) (-15.0805, -0.9612) (-15.0767, -0.9614) (-15.0729, -0.9615) (-15.0693, -0.9616) (-15.0657, -0.9617) (-15.0622, -0.9618) (-15.0588, -0.9619) (-15.0555, -0.9619) (-15.0523, -0.962) (-15.0492, -0.962) (-15.0462, -0.9621) (-15.0433, -0.9621) (-15.0404, -0.9621) (-15.0377, -0.9621) (-15.0351, -0.9621) (-15.0325, -0.9621) (-15.0301, -0.9621) (-15.0277, -0.9621) (-15.0255, -0.9621) (-15.0234, -0.962) (-15.0213, -0.962) (-15.0194, -0.962) (-15.0176, -0.9619) (-15.0159, -0.9619) (-15.0143, -0.9619) (-15.0128, -0.9618) (-15.0115, -0.9618) (-15.0102, -0.9617) (-15.0091, -0.9617) (-15.008, -0.9616) (-15.0071, -0.9616) (-15.0063, -0.9616) (-15.0058, -0.9615) (-15.0055, -0.9615) (-15.0053, -0.9615) (-15.0052, -0.9615) knots -1 -1 -1 -1 -1 -1 -0.99583333 -0.99166667 -0.9875 -0.98333333 -0.97916667 -0.975 -0.97083333 -0.96666667 -0.9625 -0.95833333 -0.95416667 -0.95 -0.94583333 -0.94166667 -0.9375 -0.93333333 -0.92916667 -0.925 -0.92083333 -0.91666667 -0.9125 -0.90833333 -0.90416667 -0.9 -0.89583333 -0.89166667 -0.8875 -0.88333333 -0.87916667 -0.875 -0.87083333 -0.86666667 -0.8625 -0.85833333 -0.85416667 -0.85 -0.84583333 -0.84166667 -0.8375 -0.83333333 -0.82916667 -0.825 -0.82083333 -0.81666667 -0.8125 -0.80833333 -0.80416667 -0.8 -0.79583333 -0.79166667 -0.7875 -0.78333333 -0.77916667 -0.775 -0.77083333 -0.76666667 -0.7625 -0.75833333 -0.75416667 -0.75 -0.74583333 -0.74166667 -0.7375 -0.73333333 -0.72916667 -0.725 -0.72083333 -0.71666667 -0.7125 -0.70833333 -0.70416667 -0.7 -0.69583333 -0.69166667 -0.6875 -0.68333333 -0.67916667 -0.675 -0.67083333 -0.66666667 -0.6625 -0.65833333 -0.65416667 -0.65 -0.64583333 -0.64166667 -0.6375 -0.63333333 -0.62916667 -0.625 -0.62083333 -0.61666667 -0.6125 -0.60833333 -0.60416667 -0.6 -0.59583333 -0.59166667 -0.5875 -0.58333333 -0.57916667 -0.575 -0.57083333 -0.56666667 -0.5625 -0.55833333 -0.55416667 -0.55 -0.54583333 -0.54166667 -0.5375 -0.53333333 -0.52916667 -0.525 -0.52083333 -0.51666667 -0.5125 -0.50833333 -0.50416667 -0.5 -0.49583333 -0.49166667 -0.4875 -0.48333333 -0.47916667 -0.475 -0.47083333 -0.46666667 -0.4625 -0.45833333 -0.45416667 -0.45 -0.44583333 -0.44166667 -0.4375 -0.43333333 -0.42916667 -0.425 -0.42083333 -0.41666667 -0.4125 -0.40833333 -0.40416667 -0.4 -0.39583333 -0.39166667 -0.3875 -0.38333333 -0.37916667 -0.375 -0.37083333 -0.36666667 -0.3625 -0.35833333 -0.35416667 -0.35 -0.34583333 -0.34166667 -0.3375 -0.33333333 -0.32916667 -0.325 -0.32083333 -0.31666667 -0.3125 -0.30833333 -0.30416667 -0.3 -0.29583333 -0.29166667 -0.2875 -0.28333333 -0.27916667 -0.275 -0.27083333 -0.26666667 -0.2625 -0.25833333 -0.25416667 -0.25 -0.24583333 -0.24166667 -0.2375 -0.23333333 -0.22916667 -0.225 -0.22083333 -0.21666667 -0.2125 -0.20833333 -0.20416667 -0.2 -0.19583333 -0.19166667 -0.1875 -0.18333333 -0.17916667 -0.175 -0.17083333 -0.16666667 -0.1625 -0.15833333 -0.15416667 -0.15 -0.14583333 -0.14166667 -0.1375 -0.13333333 -0.12916667 -0.125 -0.12083333 -0.11666667 -0.1125 -0.10833333 -0.10416667 -0.1 -0.09583333 -0.09166667 -0.0875 -0.08333333 -0.07916667 -0.075 -0.07083333 -0.06666667 -0.0625 -0.05833333 -0.05416667 -0.05 -0.04583333 -0.04166667 -0.0375 -0.03333333 -0.02916667 -0.025 -0.02083333 -0.01666667 -0.0125 -0.00833333 -0.00416667 0 0 0 0 0 0
  line L2 (-15.0052, -0.9615) -> (-15.0043, -0.9615)
  line L3 (-15.0043, -0.9615) -> (-14.7198, -0.9432)
  arc A2 (-14.7198, -0.9432) -> (-14.621, -1.9466) centre (0, 0) ccw
  line L4 (-14.621, -1.9466) -> (-14.9036, -1.9842)
  line L5 (-14.9036, -1.9842) -> (-14.9044, -1.9843)
  spline S2 degree 5 poles (-14.9044, -1.9843) (-14.9045, -1.9843) (-14.9047, -1.9844) (-14.9051, -1.9844) (-14.9056, -1.9845) (-14.9064, -1.9846) (-14.9073, -1.9848) (-14.9083, -1.9849) (-14.9094, -1.9851) (-14.9106, -1.9853) (-14.912, -1.9855) (-14.9135, -1.9858) (-14.915, -1.986) (-14.9167, -1.9863) (-14.9185, -1.9866) (-14.9204, -1.987) (-14.9224, -1.9874) (-14.9245, -1.9877) (-14.9267, -1.9882) (-14.929, -1.9886) (-14.9314, -1.9891) (-14.9339, -1.9896) (-14.9365, -1.9901) (-14.9391, -1.9906) (-14.9419, -1.9912) (-14.9448, -1.9918) (-14.9477, -1.9924) (-14.9508, -1.9931) (-14.9539, -1.9937) (-14.9571, -1.9945) (-14.9605, -1.9952) (-14.9639, -1.996) (-14.9673, -1.9968) (-14.9709, -1.9976) (-14.9746, -1.9984) (-14.9783, -1.9993) (-14.9821, -2.0002) (-14.986, -2.0012) (-14.99, -2.0021) (-14.994, -2.0031) (-14.9981, -2.0042) (-15.0023, -2.0052) (-15.0066, -2.0063) (-15.011, -2.0074) (-15.0154, -2.0086) (-15.0199, -2.0098) (-15.0245, -2.011) (-15.0291, -2.0122) (-15.0338, -2.0135) (-15.0386, -2.0148) (-15.0435, -2.0161) (-15.0484, -2.0175) (-15.0534, -2.0189) (-15.0584, -2.0204) (-15.0636, -2.0218) (-15.0688, -2.0233) (-15.074, -2.0249) (-15.0794, -2.0264) (-15.0847, -2.028) (-15.0902, -2.0297) (-15.0957, -2.0313) (-15.1013, -2.033) (-15.1069, -2.0348) (-15.1126, -2.0365) (-15.1184, -2.0383) (-15.1242, -2.0402) (-15.1301, -2.042) (-15.136, -2.0439) (-15.142, -2.0459) (-15.1481, -2.0478) (-15.1542, -2.0499) (-15.1604, -2.0519) (-15.1666, -2.054) (-15.1729, -2.0561) (-15.1792, -2.0582) (-15.1856, -2.0604) (-15.1921, -2.0626) (-15.1986, -2.0649) (-15.2051, -2.0671) (-15.2117, -2.0695) (-15.2184, -2.0718) (-15.2251, -2.0742) (-15.2318, -2.0766) (-15.2387, -2.0791) (-15.2455, -2.0816) (-15.2524, -2.0841) (-15.2594, -2.0867) (-15.2664, -2.0893) (-15.2735, -2.0919) (-15.2806, -2.0946) (-15.2877, -2.0973) (-15.2949, -2.1001) (-15.3022, -2.1028) (-15.3095, -2.1057) (-15.3168, -2.1085) (-15.3242, -2.1114) (-15.3316, -2.1143) (-15.3391, -2.1173) (-15.3466, -2.1203) (-15.3542, -2.1233) (-15.3618, -2.1264) (-15.3694, -2.1295) (-15.3771, -2.1327) (-15.3849, -2.1359) (-15.3927, -2.1391) (-15.4005, -2.1423) (-15.4083, -2.1456) (-15.4162, -2.149) (-15.4242, -2.1523) (-15.4322, -2.1558) (-15.4402, -2.1592) (-15.4483, -2.1627) (-15.4564, -2.1662) (-15.4645, -2.1698) (-15.4727, -2.1734) (-15.4809, -2.177) (-15.4892, -2.1807) (-15.4974, -2.1844) (-15.5058, -2.1881) (-15.5141, -2.1919) (-15.5226, -2.1957) (-15.531, -2.1996) (-15.5395, -2.2035) (-15.548, -2.2074) (-15.5565, -2.2114) (-15.5651, -2.2154) (-15.5737, -2.2194) (-15.5824, -2.2235) (-15.5911, -2.2276) (-15.5998, -2.2318) (-15.6085, -2.236) (-15.6173, -2.2402) (-15.6261, -2.2445) (-15.635, -2.2488) (-15.6439, -2.2532) (-15.6528, -2.2576) (-15.6617, -2.262) (-15.6707, -2.2665) (-15.6797, -2.271) (-15.6888, -2.2755) (-15.6979, -2.2801) (-15.707, -2.2847) (-15.7161, -2.2894) (-15.7253, -2.2941) (-15.7344, -2.2988) (-15.7437, -2.3036) (-15.7529, -2.3084) (-15.7622, -2.3132) (-15.7715, -2.3181) (-15.7808, -2.3231) (-15.7902, -2.328) (-15.7996, -2.333) (-15.809, -2.3381) (-15.8185, -2.3432) (-15.8279, -2.3483) (-15.8374, -2.3534) (-15.847, -2.3586) (-15.8565, -2.3639) (-15.8661, -2.3692) (-15.8757, -2.3745) (-15.8853, -2.3798) (-15.895, -2.3852) (-15.9047, -2.3907) (-15.9144, -2.3961) (-15.9241, -2.4016) (-15.9339, -2.4072) (-15.9436, -2.4128) (-15.9535, -2.4184) (-15.9633, -2.4241) (-15.9731, -2.4298) (-15.983, -2.4355) (-15.9929, -2.4413) (-16.0028, -2.4471) (-16.0128, -2.453) (-16.0227, -2.4589) (-16.0327, -2.4648) (-16.0427, -2.4708) (-16.0527, -2.4768) (-16.0628, -2.4828) (-16.0729, -2.4889) (-16.083, -2.4951) (-16.0931, -2.5012) (-16.1032, -2.5074) (-16.1134, -2.5137) (-16.1235, -2.52) (-16.1337, -2.5263) (-16.144, -2.5327) (-16.1542, -2.5391) (-16.1645, -2.5455) (-16.1747, -2.552) (-16.185, -2.5585) (-16.1953, -2.5651) (-16.2057, -2.5717) (-16.216, -2.5783) (-16.2264, -2.585) (-16.2368, -2.5917) (-16.2472, -2.5985) (-16.2576, -2.6053) (-16.268, -2.6121) (-16.2785, -2.619) (-16.289, -2.6259) (-16.2994, -2.6328) (-16.3099, -2.6398) (-16.3205, -2.6469) (-16.331, -2.6539) (-16.3416, -2.661) (-16.3521, -2.6682) (-16.3627, -2.6754) (-16.3733, -2.6826) (-16.3839, -2.6898) (-16.3946, -2.6971) (-16.4052, -2.7045) (-16.4159, -2.7119) (-16.4266, -2.7193) (-16.4373, -2.7267) (-16.448, -2.7342) (-16.4587, -2.7418) (-16.4694, -2.7494) (-16.4802, -2.757) (-16.4909, -2.7646) (-16.5017, -2.7723) (-16.5125, -2.78) (-16.5233, -2.7878) (-16.5341, -2.7956) (-16.5449, -2.8035) (-16.5558, -2.8114) (-16.5666, -2.8193) (-16.5775, -2.8272) (-16.5884, -2.8352) (-16.5993, -2.8433) (-16.6102, -2.8514) (-16.6211, -2.8595) (-16.632, -2.8676) (-16.6429, -2.8758) (-16.6539, -2.8841) (-16.6648, -2.8924) (-16.6758, -2.9007) (-16.6868, -2.909) (-16.6978, -2.9174) (-16.7088, -2.9258) (-16.7198, -2.9343) (-16.7286, -2.9411) (-16.7352, -2.9462) (-16.7396, -2.9497) (-16.7418, -2.9514) knots 0 0 0 0 0 0 0.00416667 0.00833333 0.0125 0.01666667 0.02083333 0.025 0.02916667 0.03333333 0.0375 0.04166667 0.04583333 0.05 0.05416667 0.05833333 0.0625 0.06666667 0.07083333 0.075 0.07916667 0.08333333 0.0875 0.09166667 0.09583333 0.1 0.10416667 0.10833333 0.1125 0.11666667 0.12083333 0.125 0.12916667 0.13333333 0.1375 0.14166667 0.14583333 0.15 0.15416667 0.15833333 0.1625 0.16666667 0.17083333 0.175 0.17916667 0.18333333 0.1875 0.19166667 0.19583333 0.2 0.20416667 0.20833333 0.2125 0.21666667 0.22083333 0.225 0.22916667 0.23333333 0.2375 0.24166667 0.24583333 0.25 0.25416667 0.25833333 0.2625 0.26666667 0.27083333 0.275 0.27916667 0.28333333 0.2875 0.29166667 0.29583333 0.3 0.30416667 0.30833333 0.3125 0.31666667 0.32083333 0.325 0.32916667 0.33333333 0.3375 0.34166667 0.34583333 0.35 0.35416667 0.35833333 0.3625 0.36666667 0.37083333 0.375 0.37916667 0.38333333 0.3875 0.39166667 0.39583333 0.4 0.40416667 0.40833333 0.4125 0.41666667 0.42083333 0.425 0.42916667 0.43333333 0.4375 0.44166667 0.44583333 0.45 0.45416667 0.45833333 0.4625 0.46666667 0.47083333 0.475 0.47916667 0.48333333 0.4875 0.49166667 0.49583333 0.5 0.50416667 0.50833333 0.5125 0.51666667 0.52083333 0.525 0.52916667 0.53333333 0.5375 0.54166667 0.54583333 0.55 0.55416667 0.55833333 0.5625 0.56666667 0.57083333 0.575 0.57916667 0.58333333 0.5875 0.59166667 0.59583333 0.6 0.60416667 0.60833333 0.6125 0.61666667 0.62083333 0.625 0.62916667 0.63333333 0.6375 0.64166667 0.64583333 0.65 0.65416667 0.65833333 0.6625 0.66666667 0.67083333 0.675 0.67916667 0.68333333 0.6875 0.69166667 0.69583333 0.7 0.70416667 0.70833333 0.7125 0.71666667 0.72083333 0.725 0.72916667 0.73333333 0.7375 0.74166667 0.74583333 0.75 0.75416667 0.75833333 0.7625 0.76666667 0.77083333 0.775 0.77916667 0.78333333 0.7875 0.79166667 0.79583333 0.8 0.80416667 0.80833333 0.8125 0.81666667 0.82083333 0.825 0.82916667 0.83333333 0.8375 0.84166667 0.84583333 0.85 0.85416667 0.85833333 0.8625 0.86666667 0.87083333 0.875 0.87916667 0.88333333 0.8875 0.89166667 0.89583333 0.9 0.90416667 0.90833333 0.9125 0.91666667 0.92083333 0.925 0.92916667 0.93333333 0.9375 0.94166667 0.94583333 0.95 0.95416667 0.95833333 0.9625 0.96666667 0.97083333 0.975 0.97916667 0.98333333 0.9875 0.99166667 0.99583333 1 1 1 1 1 1
  arc A3 (-16.7418, -2.9514) -> (-16.5969, -3.6801) centre (0, 0) ccw
  spline S3 degree 5 poles (-16.5969, -3.6801) (-16.5942, -3.6808) (-16.5888, -3.6823) (-16.5807, -3.6845) (-16.57, -3.6874) (-16.5566, -3.691) (-16.5432, -3.6946) (-16.5298, -3.6982) (-16.5165, -3.7017) (-16.5032, -3.7052) (-16.4899, -3.7086) (-16.4766, -3.712) (-16.4634, -3.7154) (-16.4502, -3.7188) (-16.437, -3.7221) (-16.4238, -3.7254) (-16.4107, -3.7287) (-16.3976, -3.7319) (-16.3845, -3.7351) (-16.3714, -3.7383) (-16.3584, -3.7414) (-16.3454, -3.7445) (-16.3324, -3.7476) (-16.3194, -3.7506) (-16.3065, -3.7536) (-16.2936, -3.7566) (-16.2807, -3.7596) (-16.2679, -3.7625) (-16.2551, -3.7654) (-16.2423, -3.7683) (-16.2295, -3.7711) (-16.2168, -3.7739) (-16.2041, -3.7766) (-16.1914, -3.7794) (-16.1788, -3.7821) (-16.1661, -3.7848) (-16.1536, -3.7874) (-16.141, -3.79) (-16.1285, -3.7926) (-16.116, -3.7952) (-16.1035, -3.7977) (-16.0911, -3.8002) (-16.0786, -3.8027) (-16.0663, -3.8051) (-16.0539, -3.8075) (-16.0416, -3.8099) (-16.0293, -3.8122) (-16.017, -3.8146) (-16.0048, -3.8168) (-15.9926, -3.8191) (-15.9805, -3.8213) (-15.9683, -3.8235) (-15.9562, -3.8257) (-15.9441, -3.8279) (-15.9321, -3.83) (-15.9201, -3.8321) (-15.9081, -3.8341) (-15.8962, -3.8361) (-15.8843, -3.8381) (-15.8724, -3.8401) (-15.8606, -3.8421) (-15.8488, -3.844) (-15.837, -3.8459) (-15.8252, -3.8477) (-15.8135, -3.8495) (-15.8019, -3.8513) (-15.7902, -3.8531) (-15.7786, -3.8549) (-15.7671, -3.8566) (-15.7555, -3.8583) (-15.744, -3.8599) (-15.7326, -3.8616) (-15.7211, -3.8632) (-15.7097, -3.8648) (-15.6984, -3.8663) (-15.6871, -3.8678) (-15.6758, -3.8693) (-15.6645, -3.8708) (-15.6533, -3.8723) (-15.6422, -3.8737) (-15.631, -3.8751) (-15.6199, -3.8764) (-15.6089, -3.8778) (-15.5978, -3.8791) (-15.5869, -3.8804) (-15.5759, -3.8816) (-15.565, -3.8829) (-15.5541, -3.8841) (-15.5433, -3.8853) (-15.5325, -3.8864) (-15.5218, -3.8876) (-15.511, -3.8887) (-15.5004, -3.8897) (-15.4897, -3.8908) (-15.4791, -3.8918) (-15.4686, -3.8928) (-15.4581, -3.8938) (-15.4476, -3.8948) (-15.4372, -3.8957) (-15.4268, -3.8966) (-15.4164, -3.8975) (-15.4061, -3.8983) (-15.3959, -3.8992) (-15.3857, -3.9) (-15.3755, -3.9008) (-15.3653, -3.9015) (-15.3553, -3.9023) (-15.3452, -3.903) (-15.3352, -3.9037) (-15.3252, -3.9043) (-15.3153, -3.905) (-15.3054, -3.9056) (-15.2956, -3.9062) (-15.2858, -3.9068) (-15.2761, -3.9073) (-15.2664, -3.9079) (-15.2568, -3.9084) (-15.2471, -3.9089) (-15.2376, -3.9093) (-15.2281, -3.9098) (-15.2186, -3.9102) (-15.2092, -3.9106) (-15.1998, -3.911) (-15.1905, -3.9113) (-15.1812, -3.9116) (-15.172, -3.912) (-15.1628, -3.9123) (-15.1537, -3.9125) (-15.1446, -3.9128) (-15.1356, -3.913) (-15.1266, -3.9132) (-15.1177, -3.9134) (-15.1088, -3.9136) (-15.0999, -3.9137) (-15.0912, -3.9139) (-15.0824, -3.914) (-15.0738, -3.9141) (-15.0651, -3.9141) (-15.0565, -3.9142) (-15.048, -3.9142) (-15.0396, -3.9143) (-15.0311, -3.9143) (-15.0228, -3.9142) (-15.0145, -3.9142) (-15.0062, -3.9141) (-14.998, -3.9141) (-14.9898, -3.914) (-14.9817, -3.9139) (-14.9737, -3.9138) (-14.9657, -3.9136) (-14.9578, -3.9135) (-14.9499, -3.9133) (-14.9421, -3.9131) (-14.9343, -3.9129) (-14.9266, -3.9127) (-14.919, -3.9125) (-14.9114, -3.9122) (-14.9038, -3.912) (-14.8964, -3.9117) (-14.889, -3.9114) (-14.8816, -3.9111) (-14.8743, -3.9108) (-14.8671, -3.9104) (-14.8599, -3.9101) (-14.8528, -3.9097) (-14.8457, -3.9093) (-14.8388, -3.909) (-14.8318, -3.9086) (-14.825, -3.9081) (-14.8182, -3.9077) (-14.8114, -3.9073) (-14.8047, -3.9068) (-14.7981, -3.9064) (-14.7916, -3.9059) (-14.7851, -3.9054) (-14.7787, -3.905) (-14.7723, -3.9045) (-14.7661, -3.904) (-14.7598, -3.9034) (-14.7537, -3.9029) (-14.7476, -3.9024) (-14.7416, -3.9018) (-14.7357, -3.9013) (-14.7298, -3.9007) (-14.724, -3.9002) (-14.7182, -3.8996) (-14.7126, -3.899) (-14.707, -3.8984) (-14.7015, -3.8979) (-14.696, -3.8973) (-14.6907, -3.8967) (-14.6854, -3.8961) (-14.6801, -3.8954) (-14.675, -3.8948) (-14.6699, -3.8942) (-14.6649, -3.8936) (-14.66, -3.893) (-14.6551, -3.8923) (-14.6504, -3.8917) (-14.6457, -3.8911) (-14.6411, -3.8905) (-14.6365, -3.8898) (-14.6321, -3.8892) (-14.6277, -3.8886) (-14.6234, -3.8879) (-14.6192, -3.8873) (-14.6151, -3.8867) (-14.6111, -3.8861) (-14.6071, -3.8854) (-14.6032, -3.8848) (-14.5994, -3.8842) (-14.5957, -3.8836) (-14.5921, -3.883) (-14.5886, -3.8824) (-14.5852, -3.8818) (-14.5818, -3.8812) (-14.5786, -3.8806) (-14.5754, -3.8801) (-14.5724, -3.8795) (-14.5694, -3.8789) (-14.5665, -3.8784) (-14.5637, -3.8779) (-14.5611, -3.8773) (-14.5585, -3.8768) (-14.556, -3.8763) (-14.5536, -3.8758) (-14.5513, -3.8754) (-14.5491, -3.8749) (-14.547, -3.8745) (-14.545, -3.874) (-14.5432, -3.8736) (-14.5414, -3.8733) (-14.5397, -3.8729) (-14.5382, -3.8725) (-14.5367, -3.8722) (-14.5354, -3.8719) (-14.5342, -3.8716) (-14.533, -3.8713) (-14.532, -3.8711) (-14.5312, -3.8709) (-14.5304, -3.8707) (-14.5299, -3.8706) (-14.5296, -3.8705) (-14.5294, -3.8704) (-14.5293, -3.8704) knots -1 -1 -1 -1 -1 -1 -0.99583333 -0.99166667 -0.9875 -0.98333333 -0.97916667 -0.975 -0.97083333 -0.96666667 -0.9625 -0.95833333 -0.95416667 -0.95 -0.94583333 -0.94166667 -0.9375 -0.93333333 -0.92916667 -0.925 -0.92083333 -0.91666667 -0.9125 -0.90833333 -0.90416667 -0.9 -0.89583333 -0.89166667 -0.8875 -0.88333333 -0.87916667 -0.875 -0.87083333 -0.86666667 -0.8625 -0.85833333 -0.85416667 -0.85 -0.84583333 -0.84166667 -0.8375 -0.83333333 -0.82916667 -0.825 -0.82083333 -0.81666667 -0.8125 -0.80833333 -0.80416667 -0.8 -0.79583333 -0.79166667 -0.7875 -0.78333333 -0.77916667 -0.775 -0.77083333 -0.76666667 -0.7625 -0.75833333 -0.75416667 -0.75 -0.74583333 -0.74166667 -0.7375 -0.73333333 -0.72916667 -0.725 -0.72083333 -0.71666667 -0.7125 -0.70833333 -0.70416667 -0.7 -0.69583333 -0.69166667 -0.6875 -0.68333333 -0.67916667 -0.675 -0.67083333 -0.66666667 -0.6625 -0.65833333 -0.65416667 -0.65 -0.64583333 -0.64166667 -0.6375 -0.63333333 -0.62916667 -0.625 -0.62083333 -0.61666667 -0.6125 -0.60833333 -0.60416667 -0.6 -0.59583333 -0.59166667 -0.5875 -0.58333333 -0.57916667 -0.575 -0.57083333 -0.56666667 -0.5625 -0.55833333 -0.55416667 -0.55 -0.54583333 -0.54166667 -0.5375 -0.53333333 -0.52916667 -0.525 -0.52083333 -0.51666667 -0.5125 -0.50833333 -0.50416667 -0.5 -0.49583333 -0.49166667 -0.4875 -0.48333333 -0.47916667 -0.475 -0.47083333 -0.46666667 -0.4625 -0.45833333 -0.45416667 -0.45 -0.44583333 -0.44166667 -0.4375 -0.43333333 -0.42916667 -0.425 -0.42083333 -0.41666667 -0.4125 -0.40833333 -0.40416667 -0.4 -0.39583333 -0.39166667 -0.3875 -0.38333333 -0.37916667 -0.375 -0.37083333 -0.36666667 -0.3625 -0.35833333 -0.35416667 -0.35 -0.34583333 -0.34166667 -0.3375 -0.33333333 -0.32916667 -0.325 -0.32083333 -0.31666667 -0.3125 -0.30833333 -0.30416667 -0.3 -0.29583333 -0.29166667 -0.2875 -0.28333333 -0.27916667 -0.275 -0.27083333 -0.26666667 -0.2625 -0.25833333 -0.25416667 -0.25 -0.24583333 -0.24166667 -0.2375 -0.23333333 -0.22916667 -0.225 -0.22083333 -0.21666667 -0.2125 -0.20833333 -0.20416667 -0.2 -0.19583333 -0.19166667 -0.1875 -0.18333333 -0.17916667 -0.175 -0.17083333 -0.16666667 -0.1625 -0.15833333 -0.15416667 -0.15 -0.14583333 -0.14166667 -0.1375 -0.13333333 -0.12916667 -0.125 -0.12083333 -0.11666667 -0.1125 -0.10833333 -0.10416667 -0.1 -0.09583333 -0.09166667 -0.0875 -0.08333333 -0.07916667 -0.075 -0.07083333 -0.06666667 -0.0625 -0.05833333 -0.05416667 -0.05 -0.04583333 -0.04166667 -0.0375 -0.03333333 -0.02916667 -0.025 -0.02083333 -0.01666667 -0.0125 -0.00833333 -0.00416667 0 0 0 0 0 0
  line L6 (-14.5293, -3.8704) -> (-14.5284, -3.8702)
  line L7 (-14.5284, -3.8702) -> (-14.253, -3.7968)
  arc A4 (-14.253, -3.7968) -> (-13.9603, -4.7616) centre (0, 0) ccw
  line L8 (-13.9603, -4.7616) -> (-14.2301, -4.8536)
  line L9 (-14.2301, -4.8536) -> (-14.2309, -4.8539)